Autodesk Fusion 360 part; units mm, degrees
(part 4 of 4)
sketch "Sketch16" plane through (0, 0, 59.6448) normal (0, 0, 1) x (1, 0, 0)
  line L0 (-120.231, 7.5) -> (-97.391, 7.5)
  line L1 (-97.391, 7.5) -> (-97.391, 3.5)
  line L2 (-97.391, 3.5) -> (-89.391, 3.5)
  line L3 (-89.391, 3.5) -> (-89.391, 7.5)
  line L4 (-89.391, 7.5) -> (117.156293, 7.5)
  line L5 (117.156293, 7.5) -> (117.156293, 9.5)
  line L6 (117.156293, 9.5) -> (-120.231, 9.5)
  line L7 (-120.231, 9.5) -> (-120.231, 7.5)
  line L8 (-96.391, 6.5) -> (-90.391, 6.5)
  line L9 (-90.391, 6.5) -> (-90.391, 4)
  line L10 (-90.391, 4) -> (-96.391, 4)
  line L11 (-96.391, 4) -> (-96.391, 6.5)
  dimension "d63" = 1
  dimension "d64" = 1
  dimension "d65" = 0.5
  constraint horizontal L8
  constraint vertical L9
  constraint horizontal L10
  constraint vertical L11
  measures "d63" distance of L1 L11
  measures "d64" distance of L3 L9.end
  measures "d65" distance of L2 L10
extrude "Extrude11" cut sketch "Sketch16" against normal blind 7 contours L8 L9 L10 L11 picked at (-94.391, 5.666667) bodies 3
ref_plane "WorkPlane1" through (124.156293, 13.5, 21.54485) normal (1, 0, 0) x (0, 0, -1)
ref_plane "WorkPlane2" through (-0.843707, 13.5, 21.544849) normal (1, 0, 0) x (0, 0, -1)
move_body "Move3" bodies 2 to x (1, 0, 0) y (0, 1, 0) z (0, 0, 1) at (0, 0, 0)
sketch "Sketch18" plane through (122.156293, 0, 0) normal (-1, 0, 0) x (0, 0, 1)
  line L0 (-18.555101, 4) -> (61.6448, 4)
  line L1 (61.6448, 4) -> (61.6448, 22)
  line L2 (61.6448, 22) -> (-18.555101, 22)
  line L3 (-18.555101, 22) -> (-18.555101, 4)
  line L4 (61.6448, 4) -> (-19, 4)
  line L5 (-19, 4) -> (-19, 6)
  line L6 (-19, 6) -> (61.6448, 6)
  line L7 (61.6448, 6) -> (61.6448, 4)
  dimension "d96" = 2
  constraint horizontal L4
  constraint vertical L5
  constraint horizontal L6
  constraint vertical L7
  constraint coincident L0.end L1.start
  measures "d96" distance of L4.end L5.end
extrude "Extrude12" add sketch "Sketch18" along normal blind 15 contours L0 L1 L3 L4 L6 L7 picked at (34.9115, 4.666667) bodies 2
sketch "Sketch19" plane through (-125.231, 0, 0) normal (1, 0, 0) x (0, 0, -1)
  line L0 (-61.6448, 4) -> (18.555101, 4)
  line L1 (18.555101, 4) -> (18.555101, 22)
  line L2 (18.555101, 22) -> (-61.6448, 22)
  line L3 (-61.6448, 22) -> (-61.6448, 4)
  line L4 (-61.6448, 4) -> (18.555101, 4)
  line L5 (18.555101, 4) -> (18.555101, 6)
  line L6 (18.555101, 6) -> (-61.6448, 6)
  line L7 (-61.6448, 6) -> (-61.6448, 4)
  dimension "d87" = 80.199901
  dimension "d88" = 2
  constraint horizontal L4
  constraint vertical L5
  constraint horizontal L6
  constraint vertical L7
  constraint coincident L0.start L3.end
  measures "d88" distance of L0.start L6.end
extrude "Extrude13" add sketch "Sketch19" along normal blind 20 contours L0 L1 L3 L4 L5 L6 L7 picked at (-34.9115, 5.333333) bodies 2
move_body "Move4" bodies 3 to x (1, 0, 0) y (0, 1, 0) z (0, 0, 1) at (0, 1.5, 0)
sketch "Sketch20" plane through (0, 6, 0) normal (0, 1, 0) x (-1, 0, 0)
  line L0 (-122.156293, 61.6448) -> (-122.156293, -18.555101)
  line L1 (-122.156293, -18.555101) -> (-107.156293, -18.555101)
  line L2 (-107.156293, -18.555101) -> (-107.156293, 61.6448)
  line L3 (-107.156293, 61.6448) -> (-122.156293, 61.6448)
  line L4 (-120.156293, 19.655775) -> (-107.259872, 19.655775)
  line L5 (-107.259872, 19.655775) -> (-107.259872, -16.555101)
  line L6 (-107.259872, -16.555101) -> (-120.156293, -16.555101)
  line L7 (-120.156293, -16.555101) -> (-120.156293, 19.655775)
  line L8 (-120.156293, 56.6448) -> (-120.156293, -13.555101)
  line L9 (-117.156293, -16.555101) -> (120.231, -16.555101)
  constraint horizontal L4
  constraint vertical L5
  constraint horizontal L6
  constraint vertical L7
extrude "Extrude14" cut sketch "Sketch20" against normal blind 10 contours L4 L5 L6 L7 L8 L9 picked at (-111.558679, -3.484809) bodies 2
sketch "Sketch21" plane through (0, 0, 0) normal (0, -1, 0) x (1, 0, 0)
  line L0 (107.259872, -16.555101) -> (107.259872, 19.655775)
  line L1 (107.259872, 19.655775) -> (120.156293, 19.655775)
  line L2 (120.156293, 19.655775) -> (120.156293, -16.555101)
  line L3 (120.156293, -16.555101) -> (107.259872, -16.555101)
  line L4 (-124.231, -17.555101) -> (121.156293, -17.555101)
  line L5 (121.156293, -17.555101) -> (121.156293, 60.6448)
  line L6 (-100.231, 60.6448) -> (-124.231, 60.6448)
  line L7 (115.761515, 12.339499) -> (117.156293, 12.339499)
  line L8 (120.156293, 9.339499) -> (120.156293, 4.550337)
  line L9 (117.156293, 1.550337) -> (115.761515, 1.550337)
  line L10 (112.761515, 4.550337) -> (112.761515, 9.339499)
  line L11 (116.458904, 12.339499) -> (116.458904, 1.550337) construction
  line L12 (112.761515, 6.944918) -> (120.156293, 6.944918) construction
  arc A0 (112.761515, 4.550337) -> (115.761515, 1.550337) centre (115.761515, 4.550337) ccw
  arc A1 (117.156293, 1.550337) -> (120.156293, 4.550337) centre (117.156293, 4.550337) ccw
  arc A2 (120.156293, 9.339499) -> (117.156293, 12.339499) centre (117.156293, 9.339499) ccw
  arc A3 (115.761515, 12.339499) -> (112.761515, 9.339499) centre (115.761515, 9.339499) ccw
  line L13 (-85.231, 60.6448) -> (-85.231, 48.6448)
  line L14 (-85.231, 48.6448) -> (-100.231, 48.6448)
  line L15 (-100.231, 48.6448) -> (-100.231, 60.6448)
  line L16 (-124.231, 60.6448) -> (-124.231, -17.555101)
  line L17 (121.156293, 60.6448) -> (-85.231, 60.6448)
  point P0 (112.761515, 6.944918)
  point P1 (116.458904, 1.550337)
  point P2 (120.156293, 6.944918)
  point P3 (116.458904, 12.339499)
  dimension "d93" = 3
  constraint horizontal L7
  constraint vertical L8
  constraint horizontal L9
  constraint vertical L10
  constraint tangent L9 A0
  constraint tangent L10 A0
  constraint tangent L8 A1
  constraint tangent L9 A1
  constraint equal A0 A1
  constraint tangent L7 A2
  constraint tangent L8 A2
  constraint equal A0 A2
  constraint tangent L7 A3
  constraint tangent L10 A3
  constraint equal A0 A3
  measures "d93" radius of A0
extrude "Extrude15" add sketch "Sketch21" against normal up to surface (6 mm away) contours L0 L1 L2 L3 L7 L9 L10 A0 A1 A2 A3 picked at (114.250245, -10.509776) bodies 2
sketch "Sketch26" plane through (0, 22, 0) normal (0, 1, 0) x (-1, 0, 0)
  arc A0 (-126.156293, -20.555101) -> (-124.156293, -22.555101) centre (-124.156293, -20.555101) ccw
  line L0 (-124.156293, -22.555101) -> (-45.487722, -22.555101)
  line L1 (-45.487722, -22.555101) -> (-45.487722, -18.555101)
  line L2 (-45.487722, -18.555101) -> (-122.156293, -18.555101)
  line L3 (-122.156293, -18.555101) -> (-122.156293, 61.6448)
  line L4 (-122.156293, 61.6448) -> (125.231, 61.6448)
  line L5 (125.231, 61.6448) -> (125.231, -18.555101)
  line L6 (125.231, -18.555101) -> (41.418722, -18.555101)
  line L7 (41.418722, -18.555101) -> (41.418722, -22.555101)
  line L8 (41.418722, -22.555101) -> (127.231, -22.555101)
  arc A1 (127.231, -22.555101) -> (129.231, -20.555101) centre (127.231, -20.555101) ccw
  line L9 (129.231, -20.555101) -> (129.231, 63.6448)
  arc A2 (129.231, 63.6448) -> (127.231, 65.6448) centre (127.231, 63.6448) ccw
  line L10 (127.231, 65.6448) -> (-124.156293, 65.6448)
  arc A3 (-124.156293, 65.6448) -> (-126.156293, 63.6448) centre (-124.156293, 63.6448) ccw
  line L11 (-126.156293, 63.6448) -> (-126.156293, -20.555101)
  line L12 (-107.156293, -18.555101) -> (-107.156293, -22.556327)
  line L13 (-107.156293, 61.6448) -> (-107.156293, 65.645589)
  line L14 (100.231, 5.444899) -> (100.231, 37.6448)
  line L15 (100.231, 5.444899) -> (110.231, -4.551031)
  line L16 (100.231, 37.6448) -> (110.231, 47.648872)
  line L17 (-97.156293, 2.444899) -> (-97.156293, 40.6448)
  line L18 (-97.156293, 2.444899) -> (-107.156293, -7.555101)
  line L19 (-97.156293, 2.444899) -> (-83.014158, 2.444899) construction
  line L20 (-97.156293, 40.6448) -> (-107.156293, 50.6448)
  line L21 (110.231, 47.648872) -> (110.231, 65.6448)
  line L22 (110.231, -4.551031) -> (110.231, -22.555101)
  line L23 (-107.156293, -7.555101) -> (-107.156293, -18.555101)
  line L24 (-107.156293, 50.6448) -> (-107.156293, 61.6448)
  dimension "d114" = 24
  dimension "d115" = 24
  dimension "d117" = 21
  dimension "d118" = 21
  dimension "d120" = 135
  dimension "d123" = 25
  dimension "d124" = 25
  constraint vertical L12
  constraint vertical L13
  constraint vertical L14
  constraint perpendicular L15 L16
  constraint vertical L17
  constraint horizontal L19
  constraint perpendicular L18 L20
  constraint perpendicular L8 L22
  constraint coincident L10 L21.end
  constraint perpendicular L10 L21
  measures "d114" distance of L4 L14.end
  measures "d120" angle of L18 L19
  measures "d123" distance of L3 L17
  measures "d124" distance of L5 L14
split "Split4" by curves path "Sketch26" along L22 L15 L14 L16 L21 L12 L23 L18 L17 L20 L24 bodies 2 makes body 4 at (-119.564333, 0, 12.846223) makes body 5 at (48.222333, 4, 25.520203)
extrude "Extrude22" cut 2 faces at (-120.231, 6, 12.846223) (115.905042, 6, 41.452665) along direction (0, 1, 0) up to surface end surface through (0, 4, 0) normal (0, 1, 0) offset 0 on bodies 2 4 bodies 2 4
sketch "Sketch33" plane through (0, 6, 0) normal (0, 1, 0) x (-1, 0, 0)
  line L0 (110.231, 47.648872) -> (110.231, 61.6448)
  line L1 (110.231, 61.6448) -> (105.231, 61.6448)
  line L2 (105.231, 61.6448) -> (105.231, 42.646836)
  line L3 (105.231, 42.646836) -> (110.231, 47.648872)
extrude "Extrude23" cut sketch "Sketch33" 1 faces at (-106.897667, 6, -7.553066) along normal up to surface contours L0 L1 L2 L3 picked at (106.897667, 50.646836) end surface through (0, 4, 0) normal (0, 1, 0) offset 0 on bodies 5 bodies 5
hidden bodies 1
equation "d6 = d8"
equation "d7 = d8"
equation "d9 = d8"
equation "d19 = d18"
equation "d115 = d114"
named bodies: "Plate", "Left Split", "PCB", "Right Split", "Case"
